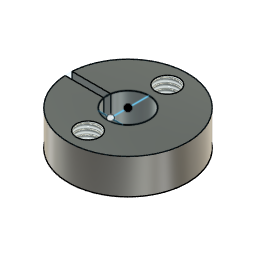
6mm D shaft nub (Autodesk Fusion 360 design; units mm, degrees)
Autodesk Fusion 360 part; units mm, degrees
note: some values were not read from the file. Set by a fixed rule: which sketch regions a step uses.
sketch "Sketch1" plane through (0, 0, 0) normal (0, 0, 1) x (1, 0, 0)
  circle A0 centre (0, 0) radius 8.5
  dimension "d1" = 17
  constraint coincident A0.centre origin
  measures "d1" diameter of A0
extrude "Extrude1" add sketch "Sketch1" along normal blind 5
sketch "Sketch2" plane through (0, 0, 5) normal (0, 0, 1) x (-1, 0, 0)
  circle A0 centre (0, 0) radius 8.5
  circle A1 centre (0, 0) radius 3
  line L0 (0, -3) -> (0, 2.5)
  line L1 (1.6583, 2.5) -> (-1.6583, 2.5)
  dimension "d4" = 6
  dimension "d5" = 5.5
  constraint coincident A0.centre A1.centre
  constraint coincident A1 L0.start
  constraint vertical L0
  constraint coincident A1 L1.start
  constraint coincident A1 L1.end
  constraint perpendicular L0 L1
  measures "d4" diameter of A1
  measures "d5" distance of L0.start L0.end
extrude "Extrude2" cut sketch "Sketch2" against normal through all contours A1 L0 L1 | A1 L0 L1
sketch "Sketch3" plane through (0, 0, 5) normal (0, 0, 1) x (-1, 0, 0)
  line L0 (-1.6583, 2.5) -> (1.6583, 2.5)
  arc A0 (-1.6583, 2.5) -> (1.6583, 2.5) centre (0, 0) ccw
  circle A1 centre (0, 0) radius 8.5
  line L1 (9.2487, -0.5) -> (2.5, -0.5)
  line L2 (2.5, -0.5) -> (2.5, 0.5)
  line L3 (2.5, 0.5) -> (9.2487, 0.5)
  line L4 (9.2487, 0.5) -> (9.2487, -0.5)
  constraint horizontal L1
  constraint vertical L2
  constraint horizontal L3
  constraint vertical L4
extrude "Extrude3" cut sketch "Sketch3" against normal through all contours A0 A1 L1 L3
sketch "Sketch7" plane through (0, 0, 5) normal (0, 0, 1) x (-1, 0, 0)
  line L0 (2.958, 0.5) -> (8.4853, 0.5)
  line L1 (8.4853, -0.5) -> (2.958, -0.5)
  arc A0 (-1.6583, 2.5) -> (2.958, -0.5) centre (0, 0) ccw
  line L2 (-1.6583, 2.5) -> (1.6583, 2.5)
  arc A1 (2.958, 0.5) -> (1.6583, 2.5) centre (0, 0) ccw
  circle A2 centre (5.7029, 0) radius 8.001
  line L3 (5.7029, 0) -> (0.0453, -5.6576)
  line L4 (5.7029, 0) -> (0.0453, 5.6576)
  line L5 (10, 0) -> (2.5113, 0)
  circle A3 centre (0.0453, -5.6576) radius 0.6892
  circle A4 centre (0.0453, 5.6576) radius 0.8487
  arc A5 (8.4853, 0.5) -> (8.4853, -0.5) centre (0, 0) ccw
  dimension "d17" = 16.002
  dimension "d18" = 45
  constraint coincident A2.centre L3.start
  constraint coincident A2 L3.end
  constraint coincident A2 L4.end
  constraint perpendicular L3 L4
  constraint coincident L3.end A3.centre
  constraint coincident L4.end A4.centre
  measures "d17" diameter of A2
  measures "d18" angle of L3 L5
hole "Hole2" at (-0.0453, -5.6576, 5) at (-0.0453, 5.6576, 5) direction (0, 0, -1) diameter 3.332 end through all
thread "Thread2" "ISO Metric profile 4.0 M4x0.7 6H" thread offset 0 thread depth 10
sketch "Sketch8" plane through (0, 0, 0) normal (0, 0, 1) x (1, 0, 0)
